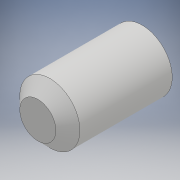
# Autodesk Inventor part: Pion croix
Saved by Autodesk Inventor 2018 (Build 220112000, 112)
## iProperties
Created: 2018-03-19
Part Number: Pion croix
Material: Générique
Document SubType Name: Modeling
Designer: Youri
Density: 1 g/cm^3
Appearance: Par défaut
Author: Youri
Autodesk Inventor part; units mm, degrees
ref_plane "YZ Plane" through (0, 0, 0) normal (1, 0, 0) x (0, 1, 0)
ref_plane "XZ Plane" through (0, 0, 0) normal (0, 1, 0) x (-1, 0, 0)
ref_plane "XY Plane" through (0, 0, 0) normal (0, 0, 1) x (1, 0, 0)
sketch "Esquisse1" plane through (0, 0, 0) normal (0, 1, 0) x (-1, 0, 0)
  circle A0 centre (0, 0) radius 7.5
  dimension "d0" = 15
  constraints: 1 centre point, 1 coincident
  measures "d0" diameter of A0
extrude "Extrusion1" add sketch "Esquisse1" along normal blind 26
chamfer "Chanfrein1" distance 3 angle 45 1 edges at (7.5, 0, 0)
sketch "Esquisse2" plane through (0, 26, 0) normal (0, 1, 0) x (1, 0, 0)
  line L0 (6, -1) -> (6, 1)
  line L1 (-6, 1) -> (-6, -1)
  line L2 (-1, -6) -> (1, -6)
  line L3 (1, 6) -> (-1, 6)
  circle A0 centre (0, 0) radius 7.5 projected
  line L4 (-1, 6) -> (-1, 1)
  line L5 (-1, -1) -> (-1, -6)
  line L6 (1, -6) -> (1, -1)
  line L7 (1, 1) -> (1, 6)
  line L8 (6, 1) -> (1, 1)
  line L9 (-1, 1) -> (-6, 1)
  line L10 (-6, -1) -> (-1, -1)
  line L11 (1, -1) -> (6, -1)
  circle A1 centre (0, 0) radius 4.5 projected
  dimension "d6" = 6
  dimension "d7" = 6
  dimension "d8" = 6
  dimension "d9" = 6
  dimension "d16" = 1
  dimension "d17" = 1
  dimension "d18" = 1
  dimension "d19" = 1
  dimension "d20" = 1
  dimension "d21" = 1
  dimension "d22" = 1
  dimension "d23" = 1
  constraints: 24 end point, 12 perpendicular, 1 horizontal, 1 vertical
  measures "d6" distance from line of L1 A0.centre
  measures "d7" distance from line of A0.centre L2
  measures "d8" distance from line of A0.centre L3
  measures "d9" distance from line of A0.centre L0
  measures "d16" distance from line of point (0, 0) L11
  measures "d17" distance from line of L8 point (0, 0)
  measures "d18" distance from line of L10 point (0, 0)
  measures "d19" distance from line of L9 point (0, 0)
  measures "d20" distance from line of L4 A1.centre
  measures "d21" distance from line of L7 point (0, 0)
  measures "d22" distance from line of L6 A0.centre
  measures "d23" distance from line of L5 point (0, 0)
extrude "Extrusion2" cut sketch "Esquisse2" against normal blind 2 contours L11 A1 L8 L0 | L11 L6 A1 L5 L10 L9 L4 L7 L8 | L6 L2 L5 A1 | A1 L4 L3 L7 | L10 L1 L9 A1
sketch "Esquisse3" plane through (0, 24, 0) normal (0, 1, 0) x (1, 0, 0)
  point P0 (0, 0)
